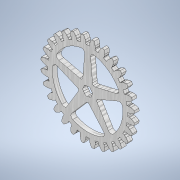
# Autodesk Inventor part: ｍ2歯数28ギア_6甲
Saved by Autodesk Inventor 2020.2 (Build 242310000, 310)
## iProperties
Created: 2020-02-11
Part Number: ｍ2歯数28ギア_6甲
Material: アルミニウム 7075
Document SubType Name: Modeling
Designer: aoyam
Density: 2.81 g/cm^3
Appearance: サテン - ブラシ仕上げ 重厚
Author: aoyam
Autodesk Inventor part; units mm, degrees
(part 1 of 3)
ref_plane "YZ Plane" through (0, 0, 0) normal (1, 0, 0) x (0, 1, 0)
ref_plane "XZ Plane" through (0, 0, 0) normal (0, 1, 0) x (-1, 0, 0)
ref_plane "XY Plane" through (0, 0, 0) normal (0, 0, 1) x (1, 0, 0)
sketch "スケッチ1" plane through (0, 0, 0) normal (0, 0, 1) x (1, 0, 0)
  arc A0 (149.6408, 131.6584) -> (149.5836, 131.2891) centre (152.0659, 131.0938) ccw
  arc A1 (150.0089, 132.8103) -> (149.6408, 131.6584) centre (156.3128, 130.1608) ccw
  arc A2 (151.1316, 134.8844) -> (150.0089, 132.8103) centre (160.8866, 128.2633) ccw
  arc A3 (147.4164, 131.2891) -> (147.3592, 131.6584) centre (144.9341, 131.0938) ccw
  arc A4 (147.3592, 131.6584) -> (146.9911, 132.8103) centre (140.6872, 130.1608) ccw
  arc A5 (146.9911, 132.8103) -> (145.8684, 134.8844) centre (136.1134, 128.2633) ccw
  arc A6 (149.5502, 130.4784) -> (147.4498, 130.4784) centre (148.5, 105) ccw
  arc A7 (145.8684, 134.8844) -> (144.4157, 134.7207) centre (148.5, 105) ccw
  line L0 (149.5502, 130.4784) -> (149.5836, 131.2891)
  line L1 (147.4498, 130.4784) -> (147.4164, 131.2891)
  line L2 (198.5, 135) -> (268.5, 135)
  line L3 (198.5, 127) -> (268.5, 127)
  line L4 (198.5, 119) -> (268.5, 119)
  line L5 (198.5, 111) -> (268.5, 111)
  line L6 (198.5, 103) -> (268.5, 103)
  line L7 (198.5, 95) -> (268.5, 95)
  line L8 (198.5, 87) -> (268.5, 87)
  line L9 (198.5, 79) -> (268.5, 79)
  line L10 (198.5, 71) -> (268.5, 71)
  line L11 (198.5, 63) -> (268.5, 63)
  line L12 (198.5, 55) -> (268.5, 55)
  line L13 (198.5, 47) -> (268.5, 47)
  line L14 (198.5, 39) -> (268.5, 39)
  line L15 (198.5, 135) -> (198.5, 39)
  line L16 (268.5, 135) -> (268.5, 39)
  line L17 (233.5, 127) -> (233.5, 39)
  arc A8 (144.4157, 134.7207) -> (143.7827, 132.4488) centre (155.3995, 130.4363) ccw
  arc A9 (143.7827, 132.4488) -> (143.6801, 131.2439) centre (150.5181, 131.2684) ccw
  arc A10 (143.6801, 131.2439) -> (143.7066, 130.8711) centre (146.1701, 131.2331) ccw
  line L18 (143.8544, 130.0733) -> (143.7066, 130.8711)
  arc A11 (143.8544, 130.0733) -> (141.8067, 129.6059) centre (148.5, 105) ccw
  line L19 (141.8067, 129.6059) -> (141.5937, 130.3888)
  arc A12 (141.5937, 130.3888) -> (141.4558, 130.7362) centre (139.217, 129.6461) ccw
  arc A13 (141.4558, 130.7362) -> (140.8405, 131.7773) centre (135.2843, 127.7914) ccw
  arc A14 (140.8405, 131.7773) -> (139.2845, 133.5495) centre (131.2474, 124.9238) ccw
  arc A15 (139.2845, 133.5495) -> (137.9046, 133.0667) centre (148.5, 105) ccw
  arc A16 (137.9046, 133.0667) -> (137.7931, 130.7109) centre (149.5664, 131.3339) ccw
  arc A17 (137.7931, 130.7109) -> (137.9612, 129.5133) centre (144.6222, 131.0589) ccw
  arc A18 (137.9612, 129.5133) -> (138.0699, 129.1558) centre (140.3911, 130.0569) ccw
  line L20 (138.3915, 128.4109) -> (138.0699, 129.1558)
  arc A19 (138.3915, 128.4109) -> (136.4992, 127.4996) centre (148.5, 105) ccw
  line L21 (136.4992, 127.4996) -> (136.1173, 128.2155)
  arc A20 (136.1173, 128.2155) -> (135.9056, 128.5234) centre (133.9655, 126.9625) ccw
  arc A21 (135.9056, 128.5234) -> (135.0741, 129.4015) centre (130.5441, 124.2792) ccw
  arc A22 (135.0741, 129.4015) -> (133.1627, 130.7831) centre (127.2465, 120.5852) ccw
  arc A23 (133.1627, 130.7831) -> (131.9249, 130.0053) centre (148.5, 105) ccw
  arc A24 (131.9249, 130.0053) -> (132.3403, 127.6838) centre (143.6798, 130.9109) ccw
  arc A25 (132.3403, 127.6838) -> (132.7707, 126.5536) centre (138.9208, 129.5427) ccw
  arc A26 (132.7707, 126.5536) -> (132.9562, 126.2292) centre (135.0187, 127.6243) ccw
  line L22 (133.4356, 125.5746) -> (132.9562, 126.2292)
  arc A27 (133.4356, 125.5746) -> (131.7934, 124.265) centre (148.5, 105) ccw
  line L23 (131.7934, 124.265) -> (131.2618, 124.878)
  arc A28 (131.2618, 124.878) -> (130.9869, 125.1311) centre (129.4428, 123.1776) ccw
  arc A29 (130.9869, 125.1311) -> (129.9808, 125.8022) centre (126.7042, 119.8003) ccw
  arc A30 (129.9808, 125.8022) -> (127.81, 126.7238) centre (124.3113, 115.4651) ccw
  arc A31 (127.81, 126.7238) -> (126.7762, 125.69) centre (148.5, 105) ccw
  arc A32 (126.7762, 125.69) -> (127.6978, 123.5192) centre (138.0349, 129.1887) ccw
  arc A33 (127.6978, 123.5192) -> (128.3689, 122.5131) centre (133.6997, 126.7958) ccw
  arc A34 (128.3689, 122.5131) -> (128.622, 122.2382) centre (130.3224, 124.0572) ccw
  line L24 (129.235, 121.7066) -> (128.622, 122.2382)
  arc A35 (129.235, 121.7066) -> (127.9254, 120.0644) centre (148.5, 105) ccw
  line L25 (127.9254, 120.0644) -> (127.2708, 120.5438)
  arc A36 (127.2708, 120.5438) -> (126.9464, 120.7293) centre (125.8757, 118.4813) ccw
  arc A37 (126.9464, 120.7293) -> (125.8162, 121.1597) centre (123.9573, 114.5792) ccw
  arc A38 (125.8162, 121.1597) -> (123.4947, 121.5751) centre (122.5891, 109.8202) ccw
  arc A39 (123.4947, 121.5751) -> (122.7169, 120.3373) centre (148.5, 105) ccw
  arc A40 (122.7169, 120.3373) -> (124.0985, 118.4259) centre (132.9148, 126.2535) ccw
  arc A41 (124.0985, 118.4259) -> (124.9766, 117.5944) centre (129.2208, 122.9559) ccw
  arc A42 (124.9766, 117.5944) -> (125.2845, 117.3827) centre (126.5375, 119.5345) ccw
  line L26 (126.0004, 117.0008) -> (125.2845, 117.3827)
  arc A43 (126.0004, 117.0008) -> (125.0891, 115.1085) centre (148.5, 105) ccw
  line L27 (125.0891, 115.1085) -> (124.3442, 115.4301)
  arc A44 (124.3442, 115.4301) -> (123.9867, 115.5388) centre (123.4431, 113.1089) ccw
  arc A45 (123.9867, 115.5388) -> (122.7891, 115.7069) centre (122.4411, 108.8778) ccw
  arc A46 (122.7891, 115.7069) -> (120.4333, 115.5954) centre (122.1661, 103.9336) ccw
  arc A47 (120.4333, 115.5954) -> (119.9505, 114.2155) centre (148.5, 105) ccw
  arc A48 (119.9505, 114.2155) -> (121.7227, 112.6595) centre (128.5762, 122.2526) ccw
  arc A49 (121.7227, 112.6595) -> (122.7638, 112.0442) centre (125.7086, 118.2157) ccw
  arc A50 (122.7638, 112.0442) -> (123.1112, 111.9063) centre (123.8539, 114.283) ccw
  line L28 (123.8941, 111.6933) -> (123.1112, 111.9063)
  arc A51 (123.8941, 111.6933) -> (123.4267, 109.6456) centre (148.5, 105) ccw
  line L29 (123.4267, 109.6456) -> (122.6289, 109.7934)
  arc A52 (122.6289, 109.7934) -> (122.2561, 109.8199) centre (122.2669, 107.3299) ccw
  arc A53 (122.2561, 109.8199) -> (121.0512, 109.7173) centre (122.2316, 102.9819) ccw
  arc A54 (121.0512, 109.7173) -> (118.7793, 109.0843) centre (123.0637, 98.1005) ccw
  arc A55 (118.7793, 109.0843) -> (118.6156, 107.6316) centre (148.5, 105) ccw
  arc A56 (118.6156, 107.6316) -> (120.6897, 106.5089) centre (125.2367, 117.3866) ccw
  arc A57 (120.6897, 106.5089) -> (121.8416, 106.1408) centre (123.3392, 112.8128) ccw
  arc A58 (121.8416, 106.1408) -> (122.2109, 106.0836) centre (122.4062, 108.5659) ccw
  line L30 (123.0216, 106.0502) -> (122.2109, 106.0836)
  arc A59 (123.0216, 106.0502) -> (123.0216, 103.9498) centre (148.5, 105) ccw
  line L31 (123.0216, 103.9498) -> (122.2109, 103.9164)
  arc A60 (122.2109, 103.9164) -> (121.8416, 103.8592) centre (122.4062, 101.4341) ccw
  arc A61 (121.8416, 103.8592) -> (120.6897, 103.4911) centre (123.3392, 97.1872) ccw
  arc A62 (120.6897, 103.4911) -> (118.6156, 102.3684) centre (125.2367, 92.6134) ccw
  arc A63 (118.6156, 102.3684) -> (118.7793, 100.9157) centre (148.5, 105) ccw
  arc A64 (118.7793, 100.9157) -> (121.0512, 100.2827) centre (123.0637, 111.8995) ccw
  arc A65 (121.0512, 100.2827) -> (122.2561, 100.1801) centre (122.2316, 107.0181) ccw
  arc A66 (122.2561, 100.1801) -> (122.6289, 100.2066) centre (122.2669, 102.6701) ccw
  line L32 (123.4267, 100.3544) -> (122.6289, 100.2066)
  arc A67 (123.4267, 100.3544) -> (123.8941, 98.3067) centre (148.5, 105) ccw
  line L33 (123.8941, 98.3067) -> (123.1112, 98.0937)
  arc A68 (123.1112, 98.0937) -> (122.7638, 97.9558) centre (123.8539, 95.717) ccw
  arc A69 (122.7638, 97.9558) -> (121.7227, 97.3405) centre (125.7086, 91.7843) ccw
  arc A70 (121.7227, 97.3405) -> (119.9505, 95.7845) centre (128.5762, 87.7474) ccw
  arc A71 (119.9505, 95.7845) -> (120.4333, 94.4046) centre (148.5, 105) ccw
  arc A72 (120.4333, 94.4046) -> (122.7891, 94.2931) centre (122.1661, 106.0664) ccw
  arc A73 (122.7891, 94.2931) -> (123.9867, 94.4612) centre (122.4411, 101.1222) ccw
  arc A74 (123.9867, 94.4612) -> (124.3442, 94.5699) centre (123.4431, 96.8911) ccw
  line L34 (125.0891, 94.8915) -> (124.3442, 94.5699)
  arc A75 (125.0891, 94.8915) -> (126.0004, 92.9992) centre (148.5, 105) ccw
  line L35 (126.0004, 92.9992) -> (125.2845, 92.6173)
  arc A76 (125.2845, 92.6173) -> (124.9766, 92.4056) centre (126.5375, 90.4655) ccw
  arc A77 (124.9766, 92.4056) -> (124.0985, 91.5741) centre (129.2208, 87.0441) ccw
  arc A78 (124.0985, 91.5741) -> (122.7169, 89.6627) centre (132.9148, 83.7465) ccw
  arc A79 (122.7169, 89.6627) -> (123.4947, 88.4249) centre (148.5, 105) ccw
  arc A80 (123.4947, 88.4249) -> (125.8162, 88.8403) centre (122.5891, 100.1798) ccw
  arc A81 (125.8162, 88.8403) -> (126.9464, 89.2707) centre (123.9573, 95.4208) ccw
  arc A82 (126.9464, 89.2707) -> (127.2708, 89.4562) centre (125.8757, 91.5187) ccw
  line L36 (127.9254, 89.9356) -> (127.2708, 89.4562)
  arc A83 (127.9254, 89.9356) -> (129.235, 88.2934) centre (148.5, 105) ccw
  line L37 (129.235, 88.2934) -> (128.622, 87.7618)
  arc A84 (128.622, 87.7618) -> (128.3689, 87.4869) centre (130.3224, 85.9428) ccw
  arc A85 (128.3689, 87.4869) -> (127.6978, 86.4808) centre (133.6997, 83.2042) ccw
  arc A86 (127.6978, 86.4808) -> (126.7762, 84.31) centre (138.0349, 80.8113) ccw
  arc A87 (126.7762, 84.31) -> (127.81, 83.2762) centre (148.5, 105) ccw
  arc A88 (127.81, 83.2762) -> (129.9808, 84.1978) centre (124.3113, 94.5349) ccw
  arc A89 (129.9808, 84.1978) -> (130.9869, 84.8689) centre (126.7042, 90.1997) ccw
  arc A90 (130.9869, 84.8689) -> (131.2618, 85.122) centre (129.4428, 86.8224) ccw
  line L38 (131.7934, 85.735) -> (131.2618, 85.122)
  arc A91 (131.7934, 85.735) -> (133.4356, 84.4254) centre (148.5, 105) ccw
  line L39 (133.4356, 84.4254) -> (132.9562, 83.7708)
  arc A92 (132.9562, 83.7708) -> (132.7707, 83.4464) centre (135.0187, 82.3757) ccw
  arc A93 (132.7707, 83.4464) -> (132.3403, 82.3162) centre (138.9208, 80.4573) ccw
  arc A94 (132.3403, 82.3162) -> (131.9249, 79.9947) centre (143.6798, 79.0891) ccw
  arc A95 (131.9249, 79.9947) -> (133.1627, 79.2169) centre (148.5, 105) ccw
  arc A96 (133.1627, 79.2169) -> (135.0741, 80.5985) centre (127.2465, 89.4148) ccw
  arc A97 (135.0741, 80.5985) -> (135.9056, 81.4766) centre (130.5441, 85.7208) ccw
  arc A98 (135.9056, 81.4766) -> (136.1173, 81.7845) centre (133.9655, 83.0375) ccw
  line L40 (136.4992, 82.5004) -> (136.1173, 81.7845)
  arc A99 (136.4992, 82.5004) -> (138.3915, 81.5891) centre (148.5, 105) ccw
  line L41 (138.3915, 81.5891) -> (138.0699, 80.8442)
  arc A100 (138.0699, 80.8442) -> (137.9612, 80.4867) centre (140.3911, 79.9431) ccw
  arc A101 (137.9612, 80.4867) -> (137.7931, 79.2891) centre (144.6222, 78.9411) ccw
  arc A102 (137.7931, 79.2891) -> (137.9046, 76.9333) centre (149.5664, 78.6661) ccw
  arc A103 (137.9046, 76.9333) -> (139.2845, 76.4505) centre (148.5, 105) ccw
  arc A104 (139.2845, 76.4505) -> (140.8405, 78.2227) centre (131.2474, 85.0762) ccw
  arc A105 (140.8405, 78.2227) -> (141.4558, 79.2638) centre (135.2843, 82.2086) ccw
  arc A106 (141.4558, 79.2638) -> (141.5937, 79.6112) centre (139.217, 80.3539) ccw
  line L42 (141.8067, 80.3941) -> (141.5937, 79.6112)
  arc A107 (141.8067, 80.3941) -> (143.8544, 79.9267) centre (148.5, 105) ccw
  line L43 (143.8544, 79.9267) -> (143.7066, 79.1289)
  arc A108 (143.7066, 79.1289) -> (143.6801, 78.7561) centre (146.1701, 78.7669) ccw
  arc A109 (143.6801, 78.7561) -> (143.7827, 77.5512) centre (150.5181, 78.7316) ccw
  arc A110 (143.7827, 77.5512) -> (144.4157, 75.2793) centre (155.3995, 79.5637) ccw
  arc A111 (144.4157, 75.2793) -> (145.8684, 75.1156) centre (148.5, 105) ccw
  arc A112 (145.8684, 75.1156) -> (146.9911, 77.1897) centre (136.1134, 81.7367) ccw
  arc A113 (146.9911, 77.1897) -> (147.3592, 78.3416) centre (140.6872, 79.8392) ccw
  arc A114 (147.3592, 78.3416) -> (147.4164, 78.7109) centre (144.9341, 78.9062) ccw
  line L44 (147.4498, 79.5216) -> (147.4164, 78.7109)
  arc A115 (147.4498, 79.5216) -> (149.5502, 79.5216) centre (148.5, 105) ccw
  line L45 (149.5502, 79.5216) -> (149.5836, 78.7109)
  arc A116 (149.5836, 78.7109) -> (149.6408, 78.3416) centre (152.0659, 78.9062) ccw
  arc A117 (149.6408, 78.3416) -> (150.0089, 77.1897) centre (156.3128, 79.8392) ccw
  arc A118 (150.0089, 77.1897) -> (151.1316, 75.1156) centre (160.8866, 81.7367) ccw
  arc A119 (151.1316, 75.1156) -> (152.5843, 75.2793) centre (148.5, 105) ccw
  arc A120 (152.5843, 75.2793) -> (153.2173, 77.5512) centre (141.6005, 79.5637) ccw
  arc A121 (153.2173, 77.5512) -> (153.3199, 78.7561) centre (146.4819, 78.7316) ccw
  arc A122 (153.3199, 78.7561) -> (153.2934, 79.1289) centre (150.8299, 78.7669) ccw
  line L46 (153.1456, 79.9267) -> (153.2934, 79.1289)
  arc A123 (153.1456, 79.9267) -> (155.1933, 80.3941) centre (148.5, 105) ccw
  line L47 (155.1933, 80.3941) -> (155.4063, 79.6112)
  arc A124 (155.4063, 79.6112) -> (155.5442, 79.2638) centre (157.783, 80.3539) ccw
  arc A125 (155.5442, 79.2638) -> (156.1595, 78.2227) centre (161.7157, 82.2086) ccw
  arc A126 (156.1595, 78.2227) -> (157.7155, 76.4505) centre (165.7526, 85.0762) ccw
  arc A127 (157.7155, 76.4505) -> (159.0954, 76.9333) centre (148.5, 105) ccw
  arc A128 (159.0954, 76.9333) -> (159.2069, 79.2891) centre (147.4336, 78.6661) ccw
  arc A129 (159.2069, 79.2891) -> (159.0388, 80.4867) centre (152.3778, 78.9411) ccw
  arc A130 (159.0388, 80.4867) -> (158.9301, 80.8442) centre (156.6089, 79.9431) ccw
  line L48 (158.6085, 81.5891) -> (158.9301, 80.8442)
  arc A131 (158.6085, 81.5891) -> (160.5008, 82.5004) centre (148.5, 105) ccw
  line L49 (160.5008, 82.5004) -> (160.8827, 81.7845)
  arc A132 (160.8827, 81.7845) -> (161.0944, 81.4766) centre (163.0345, 83.0375) ccw
  arc A133 (161.0944, 81.4766) -> (161.9259, 80.5985) centre (166.4559, 85.7208) ccw
  arc A134 (161.9259, 80.5985) -> (163.8373, 79.2169) centre (169.7535, 89.4148) ccw
  arc A135 (163.8373, 79.2169) -> (165.0751, 79.9947) centre (148.5, 105) ccw
  arc A136 (165.0751, 79.9947) -> (164.6597, 82.3162) centre (153.3202, 79.0891) ccw
  arc A137 (164.6597, 82.3162) -> (164.2293, 83.4464) centre (158.0792, 80.4573) ccw
  arc A138 (164.2293, 83.4464) -> (164.0438, 83.7708) centre (161.9813, 82.3757) ccw
  line L50 (163.5644, 84.4254) -> (164.0438, 83.7708)
  arc A139 (163.5644, 84.4254) -> (165.2066, 85.735) centre (148.5, 105) ccw
  line L51 (165.2066, 85.735) -> (165.7382, 85.122)
  arc A140 (165.7382, 85.122) -> (166.0131, 84.8689) centre (167.5572, 86.8224) ccw
  arc A141 (166.0131, 84.8689) -> (167.0192, 84.1978) centre (170.2958, 90.1997) ccw
  arc A142 (167.0192, 84.1978) -> (169.19, 83.2762) centre (172.6887, 94.5349) ccw
  arc A143 (169.19, 83.2762) -> (170.2238, 84.31) centre (148.5, 105) ccw
  arc A144 (170.2238, 84.31) -> (169.3022, 86.4808) centre (158.9651, 80.8113) ccw
  arc A145 (169.3022, 86.4808) -> (168.6311, 87.4869) centre (163.3003, 83.2042) ccw
  arc A146 (168.6311, 87.4869) -> (168.378, 87.7618) centre (166.6776, 85.9428) ccw
  line L52 (167.765, 88.2934) -> (168.378, 87.7618)
  arc A147 (167.765, 88.2934) -> (169.0746, 89.9356) centre (148.5, 105) ccw
  line L53 (169.0746, 89.9356) -> (169.7292, 89.4562)
  arc A148 (169.7292, 89.4562) -> (170.0536, 89.2707) centre (171.1243, 91.5187) ccw
  arc A149 (170.0536, 89.2707) -> (171.1838, 88.8403) centre (173.0427, 95.4208) ccw
  arc A150 (171.1838, 88.8403) -> (173.5053, 88.4249) centre (174.4109, 100.1798) ccw
  arc A151 (173.5053, 88.4249) -> (174.2831, 89.6627) centre (148.5, 105) ccw
  arc A152 (174.2831, 89.6627) -> (172.9015, 91.5741) centre (164.0852, 83.7465) ccw
  arc A153 (172.9015, 91.5741) -> (172.0234, 92.4056) centre (167.7792, 87.0441) ccw
  arc A154 (172.0234, 92.4056) -> (171.7155, 92.6173) centre (170.4625, 90.4655) ccw
  line L54 (170.9996, 92.9992) -> (171.7155, 92.6173)
  arc A155 (170.9996, 92.9992) -> (171.9109, 94.8915) centre (148.5, 105) ccw
  line L55 (171.9109, 94.8915) -> (172.6558, 94.5699)
  arc A156 (172.6558, 94.5699) -> (173.0133, 94.4612) centre (173.5569, 96.8911) ccw
  arc A157 (173.0133, 94.4612) -> (174.2109, 94.2931) centre (174.5589, 101.1222) ccw
  arc A158 (174.2109, 94.2931) -> (176.5667, 94.4046) centre (174.8339, 106.0664) ccw
  arc A159 (176.5667, 94.4046) -> (177.0495, 95.7845) centre (148.5, 105) ccw
  arc A160 (177.0495, 95.7845) -> (175.2773, 97.3405) centre (168.4238, 87.7474) ccw
  arc A161 (175.2773, 97.3405) -> (174.2362, 97.9558) centre (171.2914, 91.7843) ccw
  arc A162 (174.2362, 97.9558) -> (173.8888, 98.0937) centre (173.1461, 95.717) ccw
  line L56 (173.1059, 98.3067) -> (173.8888, 98.0937)
  arc A163 (173.1059, 98.3067) -> (173.5733, 100.3544) centre (148.5, 105) ccw
  line L57 (173.5733, 100.3544) -> (174.3711, 100.2066)
  arc A164 (174.3711, 100.2066) -> (174.7439, 100.1801) centre (174.7331, 102.6701) ccw
  arc A165 (174.7439, 100.1801) -> (175.9488, 100.2827) centre (174.7684, 107.0181) ccw
  arc A166 (175.9488, 100.2827) -> (178.2207, 100.9157) centre (173.9363, 111.8995) ccw
  arc A167 (178.2207, 100.9157) -> (178.3844, 102.3684) centre (148.5, 105) ccw
  arc A168 (178.3844, 102.3684) -> (176.3103, 103.4911) centre (171.7633, 92.6134) ccw
  arc A169 (176.3103, 103.4911) -> (175.1584, 103.8592) centre (173.6608, 97.1872) ccw
  arc A170 (175.1584, 103.8592) -> (174.7891, 103.9164) centre (174.5938, 101.4341) ccw
  line L58 (173.9784, 103.9498) -> (174.7891, 103.9164)
  arc A171 (173.9784, 103.9498) -> (173.9784, 106.0502) centre (148.5, 105) ccw
  line L59 (173.9784, 106.0502) -> (174.7891, 106.0836)
  arc A172 (174.7891, 106.0836) -> (175.1584, 106.1408) centre (174.5938, 108.5659) ccw
  arc A173 (175.1584, 106.1408) -> (176.3103, 106.5089) centre (173.6608, 112.8128) ccw
  arc A174 (176.3103, 106.5089) -> (178.3844, 107.6316) centre (171.7633, 117.3866) ccw
  arc A175 (178.3844, 107.6316) -> (178.2207, 109.0843) centre (148.5, 105) ccw
  arc A176 (178.2207, 109.0843) -> (175.9488, 109.7173) centre (173.9363, 98.1005) ccw
  arc A177 (175.9488, 109.7173) -> (174.7439, 109.8199) centre (174.7684, 102.9819) ccw
  arc A178 (174.7439, 109.8199) -> (174.3711, 109.7934) centre (174.7331, 107.3299) ccw
  line L60 (173.5733, 109.6456) -> (174.3711, 109.7934)
  arc A179 (173.5733, 109.6456) -> (173.1059, 111.6933) centre (148.5, 105) ccw
  line L61 (173.1059, 111.6933) -> (173.8888, 111.9063)
  arc A180 (173.8888, 111.9063) -> (174.2362, 112.0442) centre (173.1461, 114.283) ccw
  arc A181 (174.2362, 112.0442) -> (175.2773, 112.6595) centre (171.2914, 118.2157) ccw
  arc A182 (175.2773, 112.6595) -> (177.0495, 114.2155) centre (168.4238, 122.2526) ccw
  arc A183 (177.0495, 114.2155) -> (176.5667, 115.5954) centre (148.5, 105) ccw
  arc A184 (176.5667, 115.5954) -> (174.2109, 115.7069) centre (174.8339, 103.9336) ccw
  arc A185 (174.2109, 115.7069) -> (173.0133, 115.5388) centre (174.5589, 108.8778) ccw
  arc A186 (173.0133, 115.5388) -> (172.6558, 115.4301) centre (173.5569, 113.1089) ccw
  line L62 (171.9109, 115.1085) -> (172.6558, 115.4301)
  arc A187 (171.9109, 115.1085) -> (170.9996, 117.0008) centre (148.5, 105) ccw
  line L63 (170.9996, 117.0008) -> (171.7155, 117.3827)
  arc A188 (171.7155, 117.3827) -> (172.0234, 117.5944) centre (170.4625, 119.5345) ccw
  arc A189 (172.0234, 117.5944) -> (172.9015, 118.4259) centre (167.7792, 122.9559) ccw
  arc A190 (172.9015, 118.4259) -> (174.2831, 120.3373) centre (164.0852, 126.2535) ccw
  arc A191 (174.2831, 120.3373) -> (173.5053, 121.5751) centre (148.5, 105) ccw
  arc A192 (173.5053, 121.5751) -> (171.1838, 121.1597) centre (174.4109, 109.8202) ccw
  arc A193 (171.1838, 121.1597) -> (170.0536, 120.7293) centre (173.0427, 114.5792) ccw
  arc A194 (170.0536, 120.7293) -> (169.7292, 120.5438) centre (171.1243, 118.4813) ccw
  line L64 (169.0746, 120.0644) -> (169.7292, 120.5438)
  arc A195 (169.0746, 120.0644) -> (167.765, 121.7066) centre (148.5, 105) ccw
  line L65 (167.765, 121.7066) -> (168.378, 122.2382)
  arc A196 (168.378, 122.2382) -> (168.6311, 122.5131) centre (166.6776, 124.0572) ccw
  arc A197 (168.6311, 122.5131) -> (169.3022, 123.5192) centre (163.3003, 126.7958) ccw
  arc A198 (169.3022, 123.5192) -> (170.2238, 125.69) centre (158.9651, 129.1887) ccw
  arc A199 (170.2238, 125.69) -> (169.19, 126.7238) centre (148.5, 105) ccw
  arc A200 (169.19, 126.7238) -> (167.0192, 125.8022) centre (172.6887, 115.4651) ccw
  arc A201 (167.0192, 125.8022) -> (166.0131, 125.1311) centre (170.2958, 119.8003) ccw
  arc A202 (166.0131, 125.1311) -> (165.7382, 124.878) centre (167.5572, 123.1776) ccw
  line L66 (165.2066, 124.265) -> (165.7382, 124.878)
  arc A203 (165.2066, 124.265) -> (163.5644, 125.5746) centre (148.5, 105) ccw
  line L67 (163.5644, 125.5746) -> (164.0438, 126.2292)
  arc A204 (164.0438, 126.2292) -> (164.2293, 126.5536) centre (161.9813, 127.6243) ccw
  arc A205 (164.2293, 126.5536) -> (164.6597, 127.6838) centre (158.0792, 129.5427) ccw
  arc A206 (164.6597, 127.6838) -> (165.0751, 130.0053) centre (153.3202, 130.9109) ccw
  arc A207 (165.0751, 130.0053) -> (163.8373, 130.7831) centre (148.5, 105) ccw
  arc A208 (163.8373, 130.7831) -> (161.9259, 129.4015) centre (169.7535, 120.5852) ccw
  arc A209 (161.9259, 129.4015) -> (161.0944, 128.5234) centre (166.4559, 124.2792) ccw
  arc A210 (161.0944, 128.5234) -> (160.8827, 128.2155) centre (163.0345, 126.9625) ccw
  line L68 (160.5008, 127.4996) -> (160.8827, 128.2155)
  arc A211 (160.5008, 127.4996) -> (158.6085, 128.4109) centre (148.5, 105) ccw
  line L69 (158.6085, 128.4109) -> (158.9301, 129.1558)
  arc A212 (158.9301, 129.1558) -> (159.0388, 129.5133) centre (156.6089, 130.0569) ccw
  arc A213 (159.0388, 129.5133) -> (159.2069, 130.7109) centre (152.3778, 131.0589) ccw
  arc A214 (159.2069, 130.7109) -> (159.0954, 133.0667) centre (147.4336, 131.3339) ccw
  arc A215 (159.0954, 133.0667) -> (157.7155, 133.5495) centre (148.5, 105) ccw
  arc A216 (157.7155, 133.5495) -> (156.1595, 131.7773) centre (165.7526, 124.9238) ccw
  arc A217 (156.1595, 131.7773) -> (155.5442, 130.7362) centre (161.7157, 127.7914) ccw
  arc A218 (155.5442, 130.7362) -> (155.4063, 130.3888) centre (157.783, 129.6461) ccw
  line L70 (155.1933, 129.6059) -> (155.4063, 130.3888)
  arc A219 (155.1933, 129.6059) -> (153.1456, 130.0733) centre (148.5, 105) ccw
  line L71 (153.1456, 130.0733) -> (153.2934, 130.8711)
  arc A220 (153.2934, 130.8711) -> (153.3199, 131.2439) centre (150.8299, 131.2331) ccw
  arc A221 (153.3199, 131.2439) -> (153.2173, 132.4488) centre (146.4819, 131.2684) ccw
  arc A222 (153.2173, 132.4488) -> (152.5843, 134.7207) centre (141.6005, 130.4363) ccw
  arc A223 (152.5843, 134.7207) -> (151.1316, 134.8844) centre (148.5, 105) ccw
  circle A224 centre (148.5, 105) radius 5 construction
  circle A225 centre (148.5, 105) radius 5.6 construction
  circle A226 centre (148.5, 105) radius 25.5 construction
  arc A227 (144.2466, 127.0943) -> (152.7534, 127.0943) centre (148.5, 105) ccw
  arc A228 (144.6856, 109.8008) -> (152.3144, 109.8008) centre (148.5, 105) ccw
  line L72 (151.566, 111.1954) -> (150.3827, 124.9591)
  circle A229 centre (148.5, 105) radius 25.5 construction
  line L73 (145.434, 111.1954) -> (146.6173, 124.9591)
  arc A230 (146.6173, 124.9591) -> (144.2466, 127.0943) centre (144.6247, 125.1304) ccw
  arc A231 (152.7534, 127.0943) -> (150.3827, 124.9591) centre (152.3753, 125.1304) ccw
  arc A232 (144.6856, 109.8008) -> (145.434, 111.1954) centre (143.4414, 111.3667) ccw
  arc A233 (151.566, 111.1954) -> (152.3144, 109.8008) centre (153.5586, 111.3667) ccw
  arc A234 (128.936, 109.3772) -> (126.1727, 107.7823) centre (128.1573, 107.535) ccw
  line L74 (141.6604, 103.9986) -> (128.936, 109.3772)
  line L75 (143.5552, 109.8304) -> (130.0996, 112.9582)
  arc A235 (128.8014, 115.8727) -> (130.0996, 112.9582) centre (130.5524, 114.9063) ccw
  arc A236 (142.7554, 102.8558) -> (141.6604, 103.9986) centre (140.8817, 102.1564) ccw
  arc A237 (143.5552, 109.8304) -> (145.1129, 110.1113) centre (144.0081, 111.7784) ccw
  arc A238 (138.2915, 87.7462) -> (138.9544, 84.6252) centre (139.8029, 86.4363) ccw
  line L76 (147.3388, 98.1857) -> (138.2915, 87.7462)
  line L77 (142.378, 101.7899) -> (135.2453, 89.9594)
  arc A239 (132.0722, 89.6254) -> (135.2453, 89.9594) centre (133.5325, 90.992) ccw
  arc A240 (148.7641, 98.874) -> (147.3388, 98.1857) centre (148.8502, 96.8758) ccw
  arc A241 (142.378, 101.7899) -> (142.5922, 103.3581) centre (140.6652, 102.8226) ccw
  arc A242 (161.7547, 89.9594) -> (164.9278, 89.6254) centre (163.4675, 90.992) ccw
  line L78 (154.622, 101.7899) -> (161.7547, 89.9594)
  line L79 (149.6612, 98.1857) -> (158.7085, 87.7462)
  arc A243 (158.0456, 84.6252) -> (158.7085, 87.7462) centre (157.1971, 86.4363) ccw
  arc A244 (154.4078, 103.3581) -> (154.622, 101.7899) centre (156.3348, 102.8226) ccw
  arc A245 (149.6612, 98.1857) -> (148.2359, 98.874) centre (148.1498, 96.8758) ccw
  arc A246 (166.9004, 112.9582) -> (168.1986, 115.8727) centre (166.4476, 114.9063) ccw
  line L80 (153.4448, 109.8304) -> (166.9004, 112.9582)
  line L81 (155.3396, 103.9986) -> (168.064, 109.3772)
  arc A247 (170.8273, 107.7823) -> (168.064, 109.3772) centre (168.8427, 107.535) ccw
  arc A248 (151.8871, 110.1113) -> (153.4448, 109.8304) centre (152.9919, 111.7784) ccw
  arc A249 (155.3396, 103.9986) -> (154.2446, 102.8558) centre (156.1183, 102.1564) ccw
  line L82 (147.6679, 107.6757) -> (148.737, 107.792)
  line L83 (150.4012, 107.0584) -> (151.0365, 106.1907)
  line L84 (151.2333, 104.3828) -> (150.7995, 103.3987)
  line L85 (149.3321, 102.3243) -> (148.263, 102.208)
  line L86 (146.5988, 102.9416) -> (145.9635, 103.8093)
  line L87 (145.7667, 105.6172) -> (146.2005, 106.6013)
  line L88 (148.5, 105) -> (146.6241, 107.5621) construction
  arc A250 (147.6679, 107.6757) -> (146.2005, 106.6013) centre (147.2444, 106.7149) ccw
  arc A251 (145.7667, 105.6172) -> (145.9635, 103.8093) centre (146.387, 104.77) ccw
  arc A252 (146.5988, 102.9416) -> (148.263, 102.208) centre (147.6427, 103.0552) ccw
  arc A253 (149.3321, 102.3243) -> (150.7995, 103.3987) centre (149.7556, 103.2851) ccw
  arc A254 (151.2333, 104.3828) -> (151.0365, 106.1907) centre (150.613, 105.23) ccw
  arc A255 (150.4012, 107.0584) -> (148.737, 107.792) centre (149.3573, 106.9448) ccw
  point P0 (0, 0)
  point P1 (148.5, 137)
  point P2 (204.5, 129)
  point P3 (207, 121)
  point P4 (207, 113)
  point P5 (204.5, 105)
  point P6 (207, 97)
  point P7 (202, 89)
  point P8 (204.5, 81)
  point P9 (204.5, 73)
  point P10 (204.5, 65)
  point P11 (207, 57)
  point P12 (207, 49)
  point P13 (204.5, 41)
  point P14 (234.5, 121)
  point P15 (249.5, 113)
  point P16 (250.75, 105)
  point P17 (247, 97)
  point P18 (249.5, 89)
  point P19 (243.25, 81)
  point P20 (249.5, 73)
  point P21 (249.5, 65)
  point P22 (244.5, 57)
  point P23 (252, 49)
  point P24 (252, 41)
  point P25 (149.5, 150.5)
  point P26 (149.5, 144.5)
  point P27 (165.6875, 150.5)
  point P28 (168.875, 144.5)
  point P29 (141.3793, 136.1977)
  point P30 (134.6157, 133.831)
  point P31 (128.5483, 130.0186)
  point P32 (123.4814, 124.9517)
  point P33 (119.669, 118.8843)
  point P34 (117.3023, 112.1207)
  point P35 (116.5, 105)
  point P36 (117.3023, 97.8793)
  point P37 (119.669, 91.1157)
  point P38 (123.4814, 85.0483)
  point P39 (128.5483, 79.9814)
  point P40 (134.6157, 76.169)
  point P41 (141.3793, 73.8023)
  point P42 (148.5, 73)
  point P43 (155.6207, 73.8023)
  point P44 (162.3843, 76.169)
  point P45 (168.4517, 79.9814)
  point P46 (173.5186, 85.0483)
  point P47 (177.331, 91.1157)
  point P48 (179.6977, 97.8793)
  point P49 (180.5, 105)
  point P50 (179.6977, 112.1207)
  point P51 (177.331, 118.8843)
  point P52 (173.5186, 124.9517)
  point P53 (168.4517, 130.0186)
  point P54 (162.3843, 133.831)
  point P55 (155.6207, 136.1977)
  point P56 (173.9784, 106.0502)
  point P57 (176.3103, 106.5089)
  point P58 (175.9488, 109.7173)
  point P59 (174.7439, 109.8199)
  point P60 (174.2362, 112.0442)
  point P61 (177.0495, 114.2155)
  point P62 (171.7155, 117.3827)
  point P63 (172.9015, 118.4259)
  point P64 (174.2831, 120.3373)
  point P65 (173.5053, 121.5751)
  point P66 (169.7292, 120.5438)
  point P67 (168.6311, 122.5131)
  point P68 (170.2238, 125.69)
  point P69 (169.19, 126.7238)
  point P70 (167.0192, 125.8022)
  point P71 (166.0131, 125.1311)
  point P72 (163.5644, 125.5746)
  point P73 (163.8373, 130.7831)
  point P74 (158.9301, 129.1558)
  point P75 (159.0388, 129.5133)
  point P76 (159.2069, 130.7109)
  point P77 (159.0954, 133.0667)
  point P78 (157.7155, 133.5495)
  point P79 (155.5442, 130.7362)
  point P80 (155.1933, 129.6059)
  point P81 (153.1456, 130.0733)
  point P82 (153.2934, 130.8711)
  point P83 (153.2173, 132.4488)
  point P84 (152.5843, 134.7207)
  point P85 (149.5836, 131.2891)
  point P86 (147.4498, 130.4784)
  point P87 (147.3592, 131.6584)
  point P88 (145.8684, 134.8844)
  point P89 (144.4157, 134.7207)
  point P90 (143.7827, 132.4488)
  point P91 (141.4558, 130.7362)
  point P92 (140.8405, 131.7773)
  point P93 (137.9046, 133.0667)
  point P94 (137.9612, 129.5133)
  point P95 (133.1627, 130.7831)
  point P96 (131.9249, 130.0053)
  point P97 (132.3403, 127.6838)
  point P98 (132.7707, 126.5536)
  point P99 (131.2618, 124.878)
  point P100 (127.81, 126.7238)
  point P101 (126.7762, 125.69)
  point P102 (127.6978, 123.5192)
  point P103 (128.3689, 122.5131)
  point P104 (127.9254, 120.0644)
  point P105 (127.2708, 120.5438)
  point P106 (126.9464, 120.7293)
  point P107 (123.4947, 121.5751)
  point P108 (122.7169, 120.3373)
  point P109 (124.9766, 117.5944)
  point P110 (123.9867, 115.5388)
  point P111 (122.7891, 115.7069)
  point P112 (120.4333, 115.5954)
  point P113 (119.9505, 114.2155)
  point P114 (121.7227, 112.6595)
  point P115 (122.7638, 112.0442)
  point P116 (122.6289, 109.7934)
  point P117 (122.2561, 109.8199)
  point P118 (121.0512, 109.7173)
  point P119 (120.6897, 106.5089)
  point P120 (123.0216, 106.0502)
  point P121 (123.0216, 103.9498)
  point P122 (121.8416, 103.8592)
  point P123 (120.6897, 103.4911)
  point P124 (118.7793, 100.9157)
  point P125 (122.2561, 100.1801)
  point P126 (123.4267, 100.3544)
  point P127 (121.7227, 97.3405)
  point P128 (120.4333, 94.4046)
  point P129 (122.7891, 94.2931)
  point P130 (123.9867, 94.4612)
  point P131 (126.0004, 92.9992)
  point P132 (124.9766, 92.4056)
  point P133 (125.8162, 88.8403)
  point P134 (126.9464, 89.2707)
  point P135 (127.6978, 86.4808)
  point P136 (126.7762, 84.31)
  point P137 (127.81, 83.2762)
  point P138 (129.9808, 84.1978)
  point P139 (130.9869, 84.8689)
  point P140 (131.2618, 85.122)
  point P141 (133.4356, 84.4254)
  point P142 (132.7707, 83.4464)
  point P143 (133.1627, 79.2169)
  point P144 (135.0741, 80.5985)
  point P145 (135.9056, 81.4766)
  point P146 (136.1173, 81.7845)
  point P147 (137.9612, 80.4867)
  point P148 (137.9046, 76.9333)
  point P149 (140.8405, 78.2227)
  point P150 (141.5937, 79.6112)
  point P151 (141.8067, 80.3941)
  point P152 (143.6801, 78.7561)
  point P153 (143.7827, 77.5512)
  point P154 (144.4157, 75.2793)
  point P155 (145.8684, 75.1156)
  point P156 (146.9911, 77.1897)
  point P157 (147.3592, 78.3416)
  point P158 (147.4498, 79.5216)
  point P159 (149.5502, 79.5216)
  point P160 (149.5836, 78.7109)
  point P161 (150.0089, 77.1897)
  point P162 (151.1316, 75.1156)
  point P163 (153.2173, 77.5512)
  point P164 (153.3199, 78.7561)
  point P165 (153.1456, 79.9267)
  point P166 (157.7155, 76.4505)
  point P167 (159.2069, 79.2891)
  point P168 (160.5008, 82.5004)
  point P169 (161.0944, 81.4766)
  point P170 (161.9259, 80.5985)
  point P171 (164.2293, 83.4464)
  point P172 (165.2066, 85.735)
  point P173 (165.7382, 85.122)
  point P174 (166.0131, 84.8689)
  point P175 (169.19, 83.2762)
  point P176 (170.2238, 84.31)
  point P177 (169.3022, 86.4808)
  point P178 (168.6311, 87.4869)
  point P179 (170.0536, 89.2707)
  point P180 (174.2831, 89.6627)
  point P181 (172.9015, 91.5741)
  point P182 (172.0234, 92.4056)
  point P183 (173.0133, 94.4612)
  point P184 (174.2109, 94.2931)
  point P185 (176.5667, 94.4046)
  point P186 (177.0495, 95.7845)
  point P187 (174.2362, 97.9558)
  point P188 (173.5733, 100.3544)
  point P189 (174.3711, 100.2066)
  point P190 (174.7439, 100.1801)
  point P191 (178.2207, 100.9157)
  point P192 (176.3103, 103.4911)
  point P193 (150.9149, 103.5591)
  point P194 (148.4596, 102.1882)
  point P195 (146.0447, 103.629)
  point P196 (146.0851, 106.4409)
  point P197 (150.1695, 127.438)
  point P198 (145.3539, 110.2631)
  point P199 (146.8305, 127.438)
  dimension "d2" = 360
  dimension "d11" = 3
  dimension "d14" = 2
  dimension "d17" = 360
  dimension "d26" = 5.5
  dimension "d27" = 2.1
  dimension "d30" = 360
  constraints: 514 point on circle, 256 centre point, 178 end point, 21 point on line, 8 tangent, 4 coincident, 3 equal radius, 1268 other
  measures "d11" radial gap between concentric circles of A226 A227
  measures "d14" radius of A230
  measures "d26" distance between parallel lines of L85 L82
  measures "d27" diameter of A250
extrude "押し出し3" add sketch "スケッチ1" along normal blind 3 contours A1 A2 A223 A222 A221 A220 L71 A219 L70 A218 A217 A216 A215 A214 A213 A212 L69 A211 L68 A210 A209 A208 A207 A206 A205 A204 L67 A203 L66 A202 A201 A200 A199 A198 A197 A196 L65 A195 L64 A194 A193 A192 A191 A190 A189 A188 L63 A187 L62 A186 A185 A184 A183 A182 A181 A180 L61 A179 L60 A178 A177 A176 A175 A174 A173 A172 L59 A171 L58 A170 A169 A168 A167 A166 A165 A164 L57 A163 L56 A162 A161 A160 A159 A158 A157 A156 L55 A155 L54 A154 A153 A152 A151 A150 A149 A148 L53 A147 L52 A146 A145 A144 A143 A142 A141 A140 L51 A139 L50 A138 A137 A136 A135 A134 A133 A132 L49 A131 L48 A130 A129 A128 A127 A126 A125 A124 L47 A123 L46 A122 A121 A120 A119 A118 A117 A116 L45 A115 L44 A114 A113 A112 A111 A110 A109 A108 L43 A107 L42 A106 A105 A104 A103 A102 A101 A100 L41 A99 L40 A98 A97 A96 A95 A94 A93 A92 L39 A91 L38 A90 A89 A88 A87 A86 A85 A84 L37 A83 L36 A82 A81 A80 A79 A78 A77 A76 L35 A75 L34 A74 A73 A72 A71 A70 A69 A68 L33 A67 L32 A66 A65 A64 A63 A62 A61 A60 L31 A59 L30 A58 A57 A56 A55 A54 A53 A52 L29 A51 L28 A50 A49 A48 A47 A46 A45 A44 L27 A43 L26 A42 A41 A40 A39 A38 A37 A36 L25 A35 L24 A34 A33 A32 A31 A30 A29 A28 L23 A27 L22 A26 A25 A24 A23 A22 A21 A20 L21 A19 L20 A18 A17 A16 A15 A14 A13 A12 L19 A11 L18 A10 A9 A8 A7 A5 A4 A3 L1 A6 L0 A0 | A235 L75 A237 A232 A228 A241 A236 L74 A234 A227 | A239 L77 A241 A236 A228 A245 A240 L76 A238 A227 | A243 L79 A245 A240 A228 A249 A244 L78 A242 A227 | A247 L81 A249 A244 A228 A233 A248 L80 A246 A227